# Autodesk Inventor part: intersection_center
Saved by Autodesk Inventor 2021 (Build 250183000, 183)
## iProperties
Created: 2021-01-02
Part Number: intersection_center
Material: Generic
Document SubType Name: Modeling
Designer: Tomasz
Density: 1 g/cm^3
Appearance: Default
Author: Tomasz
Autodesk Inventor part; units mm, degrees
ref_plane "YZ Plane" through (0, 0, 0) normal (1, 0, 0) x (0, 1, 0)
ref_plane "XZ Plane" through (0, 0, 0) normal (0, 1, 0) x (-1, 0, 0)
ref_plane "XY Plane" through (0, 0, 0) normal (0, 0, 1) x (1, 0, 0)
sketch "Sketch1" plane through (0, 0, 0) normal (0, 1, 0) x (-1, 0, 0)
  line L0 (275, 0) -> (-275, 0)
  line L1 (-275, 0) -> (-275, -550)
  line L2 (-275, -550) -> (275, -550)
  line L3 (275, -550) -> (275, 0)
  line L4 (275, 0) -> (255, 0)
  line L5 (255, 0) -> (255, -20)
  line L6 (255, -20) -> (275, -20)
  line L7 (275, -20) -> (275, 0)
  line L8 (275, -550) -> (255, -550)
  line L9 (255, -550) -> (255, -530)
  line L10 (255, -530) -> (275, -530)
  line L11 (275, -530) -> (275, -550)
  line L12 (-275, 0) -> (-255, 0)
  line L13 (-255, 0) -> (-255, -20)
  line L14 (-255, -20) -> (-275, -20)
  line L15 (-275, -20) -> (-275, 0)
  line L16 (-275, -550) -> (-255, -550)
  line L17 (-255, -550) -> (-255, -530)
  line L18 (-255, -530) -> (-275, -530)
  line L19 (-275, -530) -> (-275, -550)
  point P0 (0, 0)
  point P1 (0, 0)
  dimension "d0" = 550
  dimension "d1" = 550
  dimension "d4" = 20
  dimension "d5" = 20
  dimension "d6" = 20
  dimension "d7" = 20
  dimension "d8" = 20
  dimension "d9" = 20
  dimension "d10" = 20
  dimension "d11" = 20
  constraints: 40 end point, 10 parallel, 5 horizontal, 5 perpendicular, 1 coincident, 1 midpoint
  measures "d0" distance of L2.end L1.end
  measures "d1" distance of L1.end L0.end
  measures "d4" distance of L6.end L5.end
  measures "d5" distance of L5.end L4.end
  measures "d6" distance of L9.end L10.end
  measures "d7" distance of L8.end L9.end
  measures "d8" distance of L13.end L14.end
  measures "d9" distance of L12.end L13.end
  measures "d10" distance of L18.end L17.end
  measures "d11" distance of L17.end L16.end
extrude "Extrusion1" add sketch "Sketch1" along normal blind 3
extrude "Extrusion2" add sketch "Sketch1" along normal blind 3.1 contours L3 L6 L5 L0 | L13 L14 L1 L0 | L3 L2 L9 L10 | L18 L17 L2 L1
equation "\"d0\" = track_width"
equation "\"d1\" = track_width"
equation "\"d4\" = curb_width"
equation "\"d5\" = curb_width"
equation "\"d6\" = curb_width"
equation "\"d7\" = curb_width"
equation "\"d8\" = curb_width"
equation "\"d9\" = curb_width"
equation "\"d10\" = curb_width"
equation "\"d11\" = curb_width"
equation "\"d2\" = track_height"
equation "\"d12\" = track_height + curb_height"
equation "\"track_width\" = 550"
equation "\"curb_width\" = 20"
equation "\"track_height\" = 3"
equation "\"curb_height\" = 0.1"
body "Solid1"
